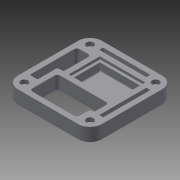
# Autodesk Inventor part: 8 pin long
Saved by Autodesk Inventor 2015 (Build 190159000, 159)
## iProperties
Created: 2014-12-11
Part Number: 8 pin long
Material: Generic
Document SubType Name: Modeling
Designer: Purple
Density: 1 g/cm^3
Appearance: Default
Author: Purple
Autodesk Inventor part; units mm, degrees
ref_plane "YZ Plane" through (0, 0, 0) normal (1, 0, 0) x (0, 1, 0)
ref_plane "XZ Plane" through (0, 0, 0) normal (0, 1, 0) x (-1, 0, 0)
sketch "Sketch1" plane through (0, 0, 0) normal (0, 1, 0) x (-1, 0, 0)
  line L0 (30, 30) -> (-30, 30)
  line L1 (-30, 30) -> (-30, -30)
  line L2 (-30, -30) -> (30, -30)
  line L3 (30, -30) -> (30, 30)
  line L4 (30, 30) -> (-30, -30) construction
  line L5 (-30, 30) -> (30, -30) construction
  point P0 (0, 0)
  dimension "d0" = 60
  dimension "d1" = 60
  constraints: 12 end point, 2 midpoint, 2 parallel, 1 horizontal, 1 perpendicular
  measures "d0" distance of L2.end L1.end
  measures "d1" distance of L0.end L1.end
extrude "Extrusion1" add sketch "Sketch1" along normal blind 10
fillet "Fillet1" radius 7 4 edges at (30, 5, 30) (30, 5, -30) (-30, 5, 30) (-30, 5, -30)
sketch "Sketch2" plane through (0, 10, 0) normal (0, 1, 0) x (1, 0, 0)
  line L0 (-30, 30) -> (30, 30)
  line L1 (30, 30) -> (30, -30)
  line L2 (30, -30) -> (-30, -30)
  line L3 (-30, -30) -> (-30, 30)
  line L4 (-30, 30) -> (30, -30) construction
  line L5 (30, 30) -> (-30, -30) construction
  line L6 (25, -25) -> (25, 25)
  line L7 (25, 25) -> (-25, 25)
  line L8 (-25, 25) -> (-25, -25)
  line L9 (-25, -25) -> (25, -25)
  circle A0 centre (25, -25) radius 2.75
  circle A1 centre (-25, -25) radius 2.75
  circle A2 centre (25, 25) radius 2.75
  circle A3 centre (-25, 25) radius 2.75
  point P0 (0, 0)
  dimension "d5" = 5
  dimension "d6" = 5.5
  dimension "d7" = 5.5
  dimension "d8" = 5.5
  dimension "d9" = 5.5
  constraints: 20 end point, 4 centre point, 4 coincident, 4 parallel, 2 midpoint, 2 perpendicular, 1 horizontal, 3 other
  measures "d5" distance between parallel lines of L1 L6
  measures "d6" diameter of A0
  measures "d7" diameter of A1
  measures "d8" diameter of A2
  measures "d9" diameter of A3
extrude "Extrusion2" cut sketch "Sketch2" against normal blind 3 contours L9 A0 L6 | L6 A0 L9 | A2 L7 L6 | L6 L7 A2 | A1 L8 L9 | L9 L8 A1 | A3 L8 L7 | L7 L8 A3
sketch "Sketch7" plane through (0, 10, 0) normal (0, 1, 0) x (1, 0, 0)
  line L0 (-23, 30) -> (23, 30)
  line L1 (30, 23) -> (30, -23)
  line L2 (23, -30) -> (-23, -30)
  line L3 (-30, -23) -> (-30, 23)
  line L4 (-30, 30) -> (30, -30) construction
  line L5 (30, 30) -> (-30, -30) construction
  arc A0 (-23, 30) -> (-30, 23) centre (-23, 23) ccw
  arc A1 (-30, -23) -> (-23, -30) centre (-23, -23) ccw
  arc A2 (23, -30) -> (30, -23) centre (23, -23) ccw
  arc A3 (30, 23) -> (23, 30) centre (23, 23) ccw
  line L6 (23, 32) -> (-23, 32)
  arc A4 (-23, 32) -> (-32, 23) centre (-23, 23) ccw
  line L7 (-32, 23) -> (-32, -23)
  arc A5 (-32, -23) -> (-23, -32) centre (-23, -23) ccw
  line L8 (-23, -32) -> (23, -32)
  arc A6 (23, -32) -> (32, -23) centre (23, -23) ccw
  line L9 (32, -23) -> (32, 23)
  arc A7 (32, 23) -> (23, 32) centre (23, 23) ccw
  point P0 (0, 0)
  dimension "d47" = 7
  dimension "d48" = 2
  constraints: 20 end point, 16 point on circle, 8 centre point, 8 point on line, 8 tangent, 4 parallel, 3 equal radius, 2 midpoint, 2 perpendicular, 1 horizontal, 7 other
  measures "d47" radius of A0
  measures "d48" distance between parallel lines of L0 L6
extrude "Extrusion6" add sketch "Sketch7" against normal blind 10
sketch "Sketch30" plane through (0, 10, 0) normal (0, 1, 0) x (1, 0, 0)
  line L0 (-25, -25) -> (25, -25)
  line L1 (25, -25) -> (25, 25)
  line L2 (25, 25) -> (-25, 25)
  line L3 (-25, 25) -> (-25, -25)
  line L4 (-25, -25) -> (25, 25) construction
  line L5 (25, -25) -> (-25, 25) construction
  line L6 (21, 21) -> (21, -21)
  line L7 (21, -21) -> (-21, -21)
  line L8 (-21, -21) -> (-21, 21)
  line L9 (-21, 21) -> (21, 21)
  line L10 (-13.4, 21) -> (-13.4, -2.8)
  line L11 (-13.4, -2.8) -> (21, -2.8)
  line L12 (19, -19) -> (-19, -19)
  line L13 (-19, -19) -> (-19, 19)
  line L14 (-11.4, 19) -> (-11.4, -0.8)
  line L15 (-11.4, -0.8) -> (19, -0.8)
  line L16 (-11.4, 19) -> (19, 19)
  line L17 (19, 19) -> (19, -0.8)
  point P0 (0, 0)
  dimension "d307" = 50
  dimension "d308" = 50
  dimension "d309" = 4
  dimension "d310" = 34.4
  dimension "d311" = 23.8
  dimension "d313" = 2
  constraints: 36 end point, 6 parallel, 4 perpendicular, 2 midpoint, 2 point on line, 1 horizontal, 1 vertical, 4 other
  measures "d307" distance of L2.end L1.end
  measures "d308" distance of L1.end L0.end
  measures "d309" distance between parallel lines of L1 L6
  measures "d310" distance of L10.start L6.start
  measures "d311" distance of L11.end L6.start
  measures "d313" distance between parallel lines of L10 L14
extrude "Extrusion28" cut sketch "Sketch30" against normal blind 2 contours L6 L11 L10 L9
sketch "Sketch31" plane through (0, 10, 0) normal (0, 1, 0) x (1, 0, 0)
  line L0 (-11.4, 19) -> (19, 19)
  line L1 (19, 19) -> (19, -0.8)
  line L2 (19, -0.8) -> (-11.4, -0.8)
  line L3 (-11.4, -0.8) -> (-11.4, 19)
  point P0 (0, 0)
  constraints: 8 end point, 2 parallel, 1 horizontal, 1 perpendicular
extrude "Extrusion29" cut sketch "Sketch31" against normal blind 8
sketch "Sketch32" plane through (0, 10, 0) normal (0, 1, 0) x (1, 0, 0)
  line L0 (32, -23) -> (32, 23) projected
  line L1 (23, 32) -> (-23, 32) projected
  line L2 (-13.4, 21) -> (21, 21) projected
  line L3 (-32, 23) -> (-32, -23) projected
  line L4 (-18, 28) -> (18, 28)
  line L5 (18, 28) -> (18, 25)
  line L6 (18, 25) -> (-18, 25)
  line L7 (-18, 25) -> (-18, 28)
  line L8 (-23, -32) -> (23, -32) projected
  line L9 (21, 21) -> (21, -2.8) projected
  line L10 (28, 18) -> (25, 18)
  line L11 (25, 18) -> (25, -18)
  line L12 (25, -18) -> (28, -18)
  line L13 (28, -18) -> (28, 18)
  line L14 (21, -2.8) -> (-13.4, -2.8) projected
  line L15 (18, -28) -> (-18, -28)
  line L16 (-18, -28) -> (-18, -6.8)
  line L17 (-18, -6.8) -> (21, -6.8)
  line L18 (21, -6.8) -> (21, -18)
  line L19 (21, -18) -> (18, -18)
  line L20 (18, -18) -> (18, -28)
  line L21 (-13.4, -2.8) -> (-13.4, 21) projected
  line L22 (-22, -18) -> (-28, -18)
  line L23 (-28, -18) -> (-28, 18)
  line L24 (-28, 18) -> (-17.4, 18)
  line L25 (-17.4, 18) -> (-17.4, -2.8)
  line L26 (-17.4, -2.8) -> (-22, -2.8)
  line L27 (-22, -2.8) -> (-22, -18)
  point P0 (0, 0)
  dimension "d318" = 14
  dimension "d319" = 4
  dimension "d320" = 4
  dimension "d321" = 4
  dimension "d322" = 14
  dimension "d323" = 4
  dimension "d324" = 14
  dimension "d325" = 4
  dimension "d326" = 14
  dimension "d327" = 4
  dimension "d328" = 14
  dimension "d329" = 4
  dimension "d330" = 4
  dimension "d331" = 4
  dimension "d332" = 14
  dimension "d333" = 4
  dimension "d334" = 14
  dimension "d335" = 4
  dimension "d336" = 14
  dimension "d337" = 4
  dimension "d338" = 4
  dimension "d339" = 4
  dimension "d341" = 4
  dimension "d342" = 14
  dimension "d343" = 14
  constraints: 40 end point, 12 perpendicular, 2 horizontal
  measures "d318" distance from line of L0 L4.end
  measures "d319" distance from line of L1 L4.end
  measures "d320" distance from line of L5.end L2
  measures "d321" distance from line of L1 L4.start
  measures "d322" distance from line of L3 L4.start
  measures "d323" distance from line of L0 L10.start
  measures "d324" distance from line of L1 L10.start
  measures "d325" distance from line of L0 L12.end
  measures "d326" distance from line of L8 L12.end
  measures "d327" distance from line of L10.end L9
  measures "d328" distance from line of L0 L15.start
  measures "d329" distance from line of L8 L15.start
  measures "d330" distance from line of L11 L18.end
  measures "d331" distance from line of L14 L17.end
  measures "d332" distance from line of L3 L15.end
  measures "d333" distance from line of L22.end L3
  measures "d334" distance from line of L8 L22.end
  measures "d335" distance from line of L16 L22.start
  measures "d336" distance from line of L8 L22.start
  measures "d337" distance from line of L17 L25.end
  measures "d338" distance from line of L21 L25.end
  measures "d339" distance from line of L21 L24.end
  measures "d341" distance from line of L3 L23.end
  measures "d342" distance from line of L1 L23.end
  measures "d343" distance from line of L1 L24.end
extrude "Extrusion30" cut sketch "Sketch32" against normal through all contours L4 L5 L6 L7 | L13 L12 L11 L10 | L15 L16 L17 L18 L19 L20 | L22 L23 L24 L25 L26 L27
fillet "Fillet9" radius 0.5 8 edges at (-18, 5, -28) (25, 5, -18) (25, 5, 18) (-18, 5, -25) (18, 5, -25) (28, 5, 18) (18, 5, -28) (28, 5, -18)
fillet "Fillet9" radius 1 10 edges at (3.8, 2, -19) (3.8, 2, 0.8) (19, 2, -9.1) (-11.4, 2, -9.1) (18, 5, 18) (21, 5, 18) (-22, 5, 2.8) (-17.4, 5, 2.8) (-22, 5, 18) (-28, 5, 18)
fillet "Fillet9" radius 2 6 edges at (-28, 5, -18) (-17.4, 5, -18) (21, 5, 6.8) (-18, 5, 28) (-18, 5, 6.8) (18, 5, 28)
ref_plane "Work Plane8" through (0, 5, 0) normal (0, 1, 0) x (1, 0, 0)
mirror "Mirror8" about plane through (0, 5, 0) normal (0, 1, 0) of "Extrusion2"
body "Solid1"
